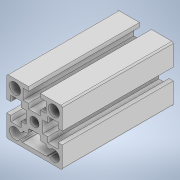
# Autodesk Inventor part: AFSF-2020-4
Saved by Autodesk Inventor 2021.1 (Build 251245010, 245A)
## iProperties
Created: 2020-11-05
Part Number: AFSF-2020-4
Material: 一般
Document SubType Name: Modeling
Designer: gisen
Density: 1 g/cm^3
Appearance: 既定
Sending System: Autodesk Inventor 2014
MC: AMD64
MC_MODEL: Intel64 Family 6 Model 94 Stepping 3, GenuineIntel
OS: Windows_NT
OS_RELEASE: 6.1
FRU: Autodesk
FORMAT: text
GUISE: transmit
KEY: AFSF-2020-4
FILE: C:\Users\AMS43\Documents\Inventor\AMS\Inventorì¬f\parasolidf\AFSF-2020-4.x_t
DATE: Mon, 29 Aug 2016 09:22:35 GMT
Author: gisen
Autodesk Inventor part; units mm, degrees
ref_plane "YZ Plane" through (0, 0, 0) normal (1, 0, 0) x (0, 1, 0)
ref_plane "XZ Plane" through (0, 0, 0) normal (0, 1, 0) x (-1, 0, 0)
ref_plane "作業平面1" through (-9.5, -10, 1000) normal (0, 0, 1) x (1, 0, 0)
sketch "スケッチ1" plane through (-9.5, -10, 1000) normal (0, 0, 1) x (1, 0, 0)
  line L0 (7.35, 18.5) -> (7.35, 20) projected
  line L1 (7.35, 20) -> (0, 20) projected
  arc A0 (0, 20) -> (-0.5, 19.5) centre (0, 19.5) ccw projected
  line L2 (-0.5, 19.5) -> (-0.5, 12.15) projected
  line L3 (-0.5, 12.15) -> (1, 12.15) projected
  line L4 (1, 12.15) -> (1, 14.15) projected
  line L5 (1, 14.15) -> (4.7, 14.15) projected
  line L6 (4.7, 14.15) -> (4.7, 12.15) projected
  line L7 (4.7, 12.15) -> (6.5, 12.15) projected
  line L8 (6.5, 12.15) -> (6.5, 7.85) projected
  line L9 (6.5, 7.85) -> (4.7, 7.85) projected
  line L10 (4.7, 7.85) -> (4.7, 5.85) projected
  line L11 (4.7, 5.85) -> (1, 5.85) projected
  line L12 (1, 5.85) -> (1, 7.85) projected
  line L13 (1, 7.85) -> (-0.5, 7.85) projected
  line L14 (-0.5, 7.85) -> (-0.5, 0.5) projected
  arc A1 (-0.5, 0.5) -> (0, 0) centre (0, 0.5) ccw projected
  line L15 (0, 0) -> (19, 0) projected
  arc A2 (19, 0) -> (19.5, 0.5) centre (19, 0.5) ccw projected
  line L16 (19.5, 0.5) -> (19.5, 7.85) projected
  line L17 (19.5, 7.85) -> (18, 7.85) projected
  line L18 (18, 7.85) -> (18, 5.85) projected
  line L19 (18, 5.85) -> (14.3, 5.85) projected
  line L20 (14.3, 5.85) -> (14.3, 7.85) projected
  line L21 (14.3, 7.85) -> (12.5, 7.85) projected
  line L22 (12.5, 7.85) -> (12.5, 12.15) projected
  line L23 (12.5, 12.15) -> (14.3, 12.15) projected
  line L24 (14.3, 12.15) -> (14.3, 14.15) projected
  line L25 (14.3, 14.15) -> (18, 14.15) projected
  line L26 (18, 14.15) -> (18, 12.15) projected
  line L27 (18, 12.15) -> (19.5, 12.15) projected
  line L28 (19.5, 12.15) -> (19.5, 19.5) projected
  arc A3 (19.5, 19.5) -> (19, 20) centre (19, 19.5) ccw projected
  line L29 (19, 20) -> (11.65, 20) projected
  line L30 (11.65, 20) -> (11.65, 18.5) projected
  line L31 (11.65, 18.5) -> (13.65, 18.5) projected
  line L32 (13.65, 18.5) -> (13.65, 14.8) projected
  line L33 (13.65, 14.8) -> (11.65, 14.8) projected
  line L34 (11.65, 14.8) -> (11.65, 13) projected
  line L35 (11.65, 13) -> (7.35, 13) projected
  line L36 (7.35, 13) -> (7.35, 14.8) projected
  line L37 (7.35, 14.8) -> (5.35, 14.8) projected
  line L38 (5.35, 14.8) -> (5.35, 18.5) projected
  line L39 (5.35, 18.5) -> (7.35, 18.5) projected
  arc A4 (11.6496, 6.4) -> (11.0496, 7) centre (11.0496, 6.4) ccw projected
  line L40 (11.6496, 6.4) -> (11.6496, 5.5) projected
  arc A5 (11.6496, 5.5) -> (11.9496, 5.2) centre (11.9496, 5.5) ccw projected
  line L41 (11.9496, 5.2) -> (13.3496, 5.2) projected
  arc A6 (13.6496, 4.9) -> (13.3496, 5.2) centre (13.3496, 4.9) ccw projected
  arc A7 (13.6496, 4.9) -> (13.7891, 4.5617) centre (13.9391, 4.8215) ccw projected
  line L42 (13.7891, 4.5617) -> (14.3769, 4.2223) projected
  arc A8 (14.3769, 4.2223) -> (15.0013, 4.3244) centre (14.6267, 4.6555) ccw projected
  arc A9 (15.0029, 1.6738) -> (15.0013, 4.3244) centre (16.5, 3) ccw projected
  arc A10 (15.0029, 1.6738) -> (14.3787, 1.7753) centre (14.6287, 1.3422) ccw projected
  line L43 (14.3787, 1.7753) -> (13.9715, 1.5402) projected
  arc A11 (13.8215, 1.5) -> (13.9715, 1.5402) centre (13.8215, 1.8) ccw projected
  line L44 (13.8215, 1.5) -> (5.1785, 1.5) projected
  arc A12 (5.0285, 1.5402) -> (5.1785, 1.5) centre (5.1785, 1.8) ccw projected
  line L45 (5.0285, 1.5402) -> (4.6213, 1.7753) projected
  arc A13 (4.6213, 1.7753) -> (3.9971, 1.6738) centre (4.3713, 1.3422) ccw projected
  arc A14 (3.9971, 4.3262) -> (3.9971, 1.6738) centre (2.5, 3) ccw projected
  arc A15 (3.9971, 4.3262) -> (4.6213, 4.2247) centre (4.3713, 4.6578) ccw projected
  line L46 (4.6213, 4.2247) -> (5.2, 4.5588) projected
  arc A16 (5.2, 4.5588) -> (5.35, 4.8187) centre (5.05, 4.8187) ccw projected
  arc A17 (5.6395, 5.1972) -> (5.35, 4.8187) centre (5.6395, 4.8972) ccw projected
  line L47 (5.6395, 5.1972) -> (7.05, 5.1972) projected
  arc A18 (7.05, 5.1972) -> (7.35, 5.4972) centre (7.05, 5.4972) ccw projected
  line L48 (7.35, 5.4972) -> (7.35, 6.4) projected
  arc A19 (7.95, 7) -> (7.35, 6.4) centre (7.95, 6.4) ccw projected
  line L49 (7.95, 7) -> (11.0496, 7) projected
  circle A20 centre (2.5, 17) radius 2 projected
  circle A21 centre (16.5, 17) radius 2 projected
  circle A22 centre (9.5, 10) radius 1.65 projected
  point P0 (9.5, 10)
extrude "押し出し1" add sketch "スケッチ1" along normal blind 40
